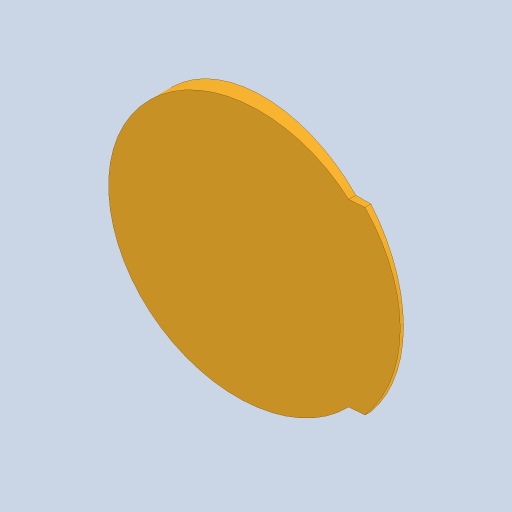
# Autodesk Inventor part: 5_grader_adapter
Saved by Autodesk Inventor 2023.1 (Build 271208000, 208)
## iProperties
Created: 2024-08-14
Part Number: 5_grader_adapter
Material: S355J2+N
Document SubType Name: Modeling
Designer: huchonms
Engineer: thingelstade
Mass: 4.32367 g
Surface Area: 9.61769 cm^2
Volume: 0.550786 cm^3
Density: 7.85 g/cm^3
Appearance: Metal (300-500 MPa)
tc_part_rev_length: 24
tc_part_rev_width: 2.25
tc_part_rev_height: 23
tc_part_rev_uom_length: mm
tc_part_rev_volume: 551
tc_part_rev_uom_volume: mm^3
tc_part_rev_mass: 0.004
tc_part_rev_uom_mass: kg
NOV_FileName: 5_grader_adapter
Author: huchonms
Revision Number: 0
Autodesk Inventor part; units mm, degrees
ref_plane "YZ Plane" through (0, 0, 0) normal (1, 0, 0) x (0, 1, 0)
ref_plane "XZ Plane" through (0, 0, 0) normal (0, 1, 0) x (-1, 0, 0)
ref_plane "XY Plane" through (0, 0, 0) normal (0, 0, 1) x (1, 0, 0)
sketch "Sketch1" plane through (0, 0, 0) normal (0, 1, 0) x (-1, 0, 0)
  arc A0 (-8.2614, -8) -> (-8.2614, 8) centre (0, 0) ccw
  line L0 (-9.6047, 8) -> (-8.2614, 8)
  arc A1 (-9.6047, 8) -> (-9.6047, -8) centre (0, 0) ccw
  line L1 (-8.2614, -8) -> (-9.6047, -8)
  constraints: 4 end point, 4 point on circle, 2 centre point
extrude "Extrusion1" add sketch "Sketch1" along normal blind 3
sketch "Sketch2" plane through (0, 0, 0) normal (0, 0, 1) x (1, 0, 0)
  line L0 (12.9833, 2.607) -> (12.9833, 0)
  line L1 (12.9833, 0) -> (-11.5556, 0)
  line L2 (-11.5556, 0) -> (12.9833, 2)
  point P0 (0, 0)
  constraints: 6 end point, 1 horizontal, 1 point on line, 1 vertical
extrude "Extrusion2" cut sketch "Sketch2" along normal mid plane 26.25
sketch "Sketch3" plane through (0, 3, 0) normal (0, 1, 0) x (1, 0, 0)
  line L0 (9.6047, 8) -> (8.2614, 8) projected
  arc A0 (8.2614, 8) -> (8.2614, -8) centre (0, 0) ccw projected
  line L1 (8.2614, -8) -> (9.6047, -8) projected
  arc A1 (9.6047, -8) -> (9.6047, 8) centre (0, 0) ccw projected
extrude "Extrusion3" cut sketch "Sketch3" against normal blind 0.75
body "Solid1"
